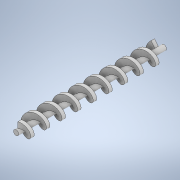
# Autodesk Inventor part: 螺旋轴2
Saved by Autodesk Inventor 2020 (Build 240168000, 168)
## iProperties
Created: 2020-06-23
Part Number: 螺旋轴2
Material: 常规
Document SubType Name: Modeling
Designer: Administrator
Density: 1 g/cm^3
Appearance: 默认
Author: Administrator
Autodesk Inventor part; units mm, degrees
ref_plane "YZ Plane" through (0, 0, 0) normal (1, 0, 0) x (0, 1, 0)
ref_plane "XZ Plane" through (0, 0, 0) normal (0, 1, 0) x (-1, 0, 0)
ref_plane "XY Plane" through (0, 0, 0) normal (0, 0, 1) x (1, 0, 0)
sketch "草图1" plane through (0, 0, 0) normal (0, 0, 1) x (1, 0, 0)
  circle A0 centre (0, 0) radius 7.5
  dimension "d0" = 15
  constraints: 1 centre point, 1 coincident
  measures "d0" diameter of A0
extrude "拉伸1" add sketch "草图1" along normal mid plane 426
sketch "草图3" plane through (0, 0, 0) normal (1, 0, 0) x (0, 1, 0)
  line L0 (0, 0) -> (0, 386.646)
  line L1 (7.5, -213) -> (7.5, 213) projected
  line L2 (7.5, 208) -> (25, 208)
  line L3 (25, 208) -> (25, 198)
  line L4 (25, 198) -> (7.5, 198)
  line L5 (7.5, 198) -> (7.5, 208)
  circle A0 centre (25, 180.5) radius 17.5 construction
  line L6 (25, 198) -> (25, 163) construction
  dimension "d3" = 50
  dimension "d4" = 5
  dimension "d5" = 35
  dimension "d6" = 10
  dimension "d7" = 35
  constraints: 12 end point, 2 parallel, 2 perpendicular, 2 point on circle, 1 centre point, 1 horizontal, 1 point on line, 1 tangent, 1 vertical
  measures "d3" diameter of L3 L0
  measures "d4" distance from line of L2 L1.end
  measures "d5" diameter of A0
  measures "d6" distance of L2.end L3.end
  measures "d7" distance of L3.end L6.end
coil "螺旋扫掠1" sketch "草图3" operation add axis through (0, 0, 0) along (0, 0, -1) pitch 45 turns 8.888889 hand right
equation "\"d8\" = d7 + d6"
